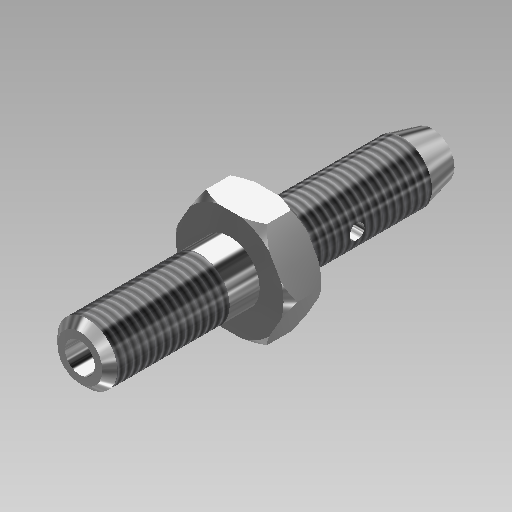
# Autodesk Inventor part: stud
Saved by Autodesk Inventor 2018.1 (Build 221171000, 171)
## iProperties
Created: 2013-08-26
Part Number: stud
Material: Generic
Document SubType Name: Modeling
Designer: Konstantin
Density: 1 g/cm^3
Appearance: Default
Mass: 0.286643 g
Surface Area: 5.38346 cm^2
Volume: 0.286643 cm^3
Author: Konstantin
Autodesk Inventor part; units mm, degrees
ref_plane "YZ Plane" through (0, 0, 0) normal (1, 0, 0) x (0, 1, 0)
ref_plane "XZ Plane" through (0, 0, 0) normal (0, 1, 0) x (-1, 0, 0)
sketch "Sketch1" plane through (0, 0, 0) normal (0, 0, 1) x (1, 0, 0)
  line L0 (2.0207, 3.5) -> (4.0415, 0)
  line L1 (4.0415, 0) -> (2.0207, -3.5)
  line L2 (2.0207, -3.5) -> (-2.0207, -3.5)
  line L3 (-2.0207, -3.5) -> (-4.0415, 0)
  line L4 (-4.0415, 0) -> (-2.0207, 3.5)
  line L5 (-2.0207, 3.5) -> (2.0207, 3.5)
  constraints: 12 end point, 2 horizontal, 4 other
extrude "Extrusion1" add sketch "Sketch1" along normal blind 2.5
sketch "Sketch2" plane through (0, 0, 2.5) normal (0, 0, 1) x (1, 0, 0)
  circle A0 centre (0, 0) radius 2
  constraints: 1 centre point, 1 coincident, 1 other
extrude "Extrusion2" add sketch "Sketch2" along normal blind 10
chamfer "Chamfer1" distance 0.5 angle 45 1 edges at (-2, 0, 12.5)
thread "Thread1" size "M4x0.5" class "6g" standard "ISO Metric profile" length 8 offset 2
sketch "Sketch3" plane through (0, 0, 0) normal (0, 0, -1) x (-1, 0, 0)
  circle A0 centre (0, 0) radius 2
  constraints: 1 centre point, 1 coincident, 1 other
extrude "Extrusion3" add sketch "Sketch3" along normal blind 11
thread "Thread2" size "M4x0.5" class "6g" standard "ISO Metric profile" length 8 offset 2
chamfer "Chamfer2" distance 0.5 distance2 2 1 edges at (2, 0, -11) measured on face at (-0.6473, -0.1595, -11)
ref_plane "Work Plane1" through (2.0207, 3.5, 0) normal (0.866, -0.5, 0) x (0, 0, 1)
sketch "Sketch5" plane through (2.0207, 3.5, 0) normal (0.866, -0.5, 0) x (0, 0, 1)
  line L0 (-0.5, 0.9514) -> (0.9514, -0.5)
  line L1 (-0.5, -0.5) -> (-0.5, 0.9514)
  line L2 (-0.5, -0.5) -> (0.9514, -0.5)
  line L3 (3, 0.9514) -> (1.5486, -0.5)
  line L4 (3, -0.5) -> (3, 0.9514)
  line L5 (3, -0.5) -> (1.5486, -0.5)
  line L6 (0, 4.0415) -> (0.9514, 4.0415) construction
  dimension "d23" = 2.0486
  constraints: 14 end point, 3 horizontal, 2 vertical, 1 parallel, 1 perpendicular, 2 other
  measures "d23" distance from line of L6.end L4
revolve "Revolution1" cut sketch "Sketch5" angle 360 about axis through (0, 0, 0) along (0, 0, 1)
sketch "Sketch6" plane through (0, 0, 12.5) normal (0, 0, 1) x (1, 0, 0)
  circle A0 centre (0, 0) radius 1
  dimension "d25" = 2
  constraints: 1 centre point, 1 coincident
  measures "d25" diameter of A0
extrude "Extrusion4" cut sketch "Sketch6" against normal blind 25
sketch "Sketch7" plane through (0, 0, 0) normal (1, 0, 0) x (0, 1, 0)
  circle A0 centre (0, -4) radius 0.5
  point P0 (0, 0)
  constraints: 1 centre point, 1 other
extrude "Extrusion5" cut sketch "Sketch7" along normal mid plane 5
body "Solid1"
